Autodesk Inventor part; units mm, degrees
(part 2 of 2)
sketch "Block3" plane through (0, 0, 0) normal (0, 0, 1) x (1, 0, 0)
  spline S0 degree 3 poles (512.2411, -949.0199) (482.4419, -902.9014) (466.6908, -849.3536) (466.6908, -794.1657) (466.6908, -740.4054) (481.691, -688.0364) (510.0715, -642.7215) (519.4139, -627.8019) (514.8946, -608.1328) (499.9744, -598.7885) (485.0506, -589.4424) (465.3833, -593.9635) (456.0413, -608.886) (421.3023, -664.3538) (402.9407, -728.4231) (402.9407, -794.1657) (402.9407, -861.6551) (422.2206, -927.1657) (458.697, -983.6183) (464.796, -993.0562) (475.039, -998.198) (485.4977, -998.198) (491.424, -998.198) (497.42, -996.5464) (502.768, -993.091) (517.5543, -983.5387) (521.7951, -963.8054) (512.2411, -949.0199) knots 0 0 0 0 1 1 1 2 2 2 3 3 3 4 4 4 5 5 5 6 6 6 7 7 7 8 8 8 9 9 9 9
  line L0 (512.2411, -949.0199) -> (482.4419, -902.9014) construction
  line L1 (482.4419, -902.9014) -> (466.6908, -849.3536) construction
  line L2 (466.6908, -849.3536) -> (466.6908, -794.1657) construction
  line L3 (466.6908, -794.1657) -> (466.6908, -740.4054) construction
  line L4 (466.6908, -740.4054) -> (481.691, -688.0364) construction
  line L5 (481.691, -688.0364) -> (510.0715, -642.7215) construction
  line L6 (510.0715, -642.7215) -> (519.4139, -627.8019) construction
  line L7 (519.4139, -627.8019) -> (514.8946, -608.1328) construction
  line L8 (514.8946, -608.1328) -> (499.9744, -598.7885) construction
  line L9 (499.9744, -598.7885) -> (485.0506, -589.4424) construction
  line L10 (485.0506, -589.4424) -> (465.3833, -593.9635) construction
  line L11 (465.3833, -593.9635) -> (456.0413, -608.886) construction
  line L12 (456.0413, -608.886) -> (421.3023, -664.3538) construction
  line L13 (421.3023, -664.3538) -> (402.9407, -728.4231) construction
  line L14 (402.9407, -728.4231) -> (402.9407, -794.1657) construction
  line L15 (402.9407, -794.1657) -> (402.9407, -861.6551) construction
  line L16 (402.9407, -861.6551) -> (422.2206, -927.1657) construction
  line L17 (422.2206, -927.1657) -> (458.697, -983.6183) construction
  line L18 (458.697, -983.6183) -> (464.796, -993.0562) construction
  line L19 (464.796, -993.0562) -> (475.039, -998.198) construction
  line L20 (475.039, -998.198) -> (485.4977, -998.198) construction
  line L21 (485.4977, -998.198) -> (491.424, -998.198) construction
  line L22 (491.424, -998.198) -> (497.42, -996.5464) construction
  line L23 (497.42, -996.5464) -> (502.768, -993.091) construction
  line L24 (502.768, -993.091) -> (517.5543, -983.5387) construction
  line L25 (517.5543, -983.5387) -> (521.7951, -963.8054) construction
  line L26 (521.7951, -963.8054) -> (512.2411, -949.0199) construction
  spline S1 degree 3 poles (319.2882, -794.1657) (319.2882, -712.6801) (342.0267, -633.2978) (385.0462, -564.6002) (394.9736, -548.7483) (390.1703, -527.8498) (374.3166, -517.9219) (358.4587, -507.988) (337.5639, -512.8013) (327.6383, -528.651) (277.8625, -608.1368) (251.5537, -699.9486) (251.5537, -794.1657) (251.5537, -890.8995) (279.1817, -984.7874) (331.4532, -1065.6794) (337.9337, -1075.7068) (348.8188, -1081.1697) (359.9295, -1081.1697) (366.2274, -1081.1697) (372.5968, -1079.4151) (378.2798, -1075.7439) (393.9893, -1065.5921) (398.4951, -1044.6277) (388.3438, -1028.9177) (343.1674, -959.0039) (319.2882, -877.8281) (319.2882, -794.1657) knots 0 0 0 0 1 1 1 2 2 2 3 3 3 4 4 4 5 5 5 6 6 6 7 7 7 8 8 8 9 9 9 9
  line L27 (319.2882, -794.1657) -> (319.2882, -712.6801) construction
  line L28 (319.2882, -712.6801) -> (342.0267, -633.2978) construction
  line L29 (342.0267, -633.2978) -> (385.0462, -564.6002) construction
  line L30 (385.0462, -564.6002) -> (394.9736, -548.7483) construction
  line L31 (394.9736, -548.7483) -> (390.1703, -527.8498) construction
  line L32 (390.1703, -527.8498) -> (374.3166, -517.9219) construction
  line L33 (374.3166, -517.9219) -> (358.4587, -507.988) construction
  line L34 (358.4587, -507.988) -> (337.5639, -512.8013) construction
  line L35 (337.5639, -512.8013) -> (327.6383, -528.651) construction
  line L36 (327.6383, -528.651) -> (277.8625, -608.1368) construction
  line L37 (277.8625, -608.1368) -> (251.5537, -699.9486) construction
  line L38 (251.5537, -699.9486) -> (251.5537, -794.1657) construction
  line L39 (251.5537, -794.1657) -> (251.5537, -890.8995) construction
  line L40 (251.5537, -890.8995) -> (279.1817, -984.7874) construction
  line L41 (279.1817, -984.7874) -> (331.4532, -1065.6794) construction
  line L42 (331.4532, -1065.6794) -> (337.9337, -1075.7068) construction
  line L43 (337.9337, -1075.7068) -> (348.8188, -1081.1697) construction
  line L44 (348.8188, -1081.1697) -> (359.9295, -1081.1697) construction
  line L45 (359.9295, -1081.1697) -> (366.2274, -1081.1697) construction
  line L46 (366.2274, -1081.1697) -> (372.5968, -1079.4151) construction
  line L47 (372.5968, -1079.4151) -> (378.2798, -1075.7439) construction
  line L48 (378.2798, -1075.7439) -> (393.9893, -1065.5921) construction
  line L49 (393.9893, -1065.5921) -> (398.4951, -1044.6277) construction
  line L50 (398.4951, -1044.6277) -> (388.3438, -1028.9177) construction
  line L51 (388.3438, -1028.9177) -> (343.1674, -959.0039) construction
  line L52 (343.1674, -959.0039) -> (319.2882, -877.8281) construction
  line L53 (319.2882, -877.8281) -> (319.2882, -794.1657) construction
  spline S2 degree 3 poles (1624.0756, -517.9219) (1608.2155, -527.8479) (1603.4145, -548.7464) (1613.3442, -564.6002) (1656.3632, -633.3018) (1679.1022, -712.6859) (1679.1022, -794.1657) (1679.1022, -877.824) (1655.2189, -958.9999) (1610.0371, -1028.9177) (1599.889, -1044.6277) (1604.3952, -1065.5921) (1620.1065, -1075.7439) (1625.7877, -1079.4168) (1632.1535, -1081.1697) (1638.4568, -1081.1697) (1649.5617, -1081.1697) (1660.4485, -1075.7068) (1666.9313, -1065.6794) (1719.2028, -984.7839) (1746.8372, -890.896) (1746.8372, -794.1657) (1746.8372, -699.9567) (1720.5256, -608.1423) (1670.7521, -528.651) (1660.8224, -512.799) (1639.9199, -507.9958) (1624.0756, -517.9219) knots 0 0 0 0 1 1 1 2 2 2 3 3 3 4 4 4 5 5 5 6 6 6 7 7 7 8 8 8 9 9 9 9
  line L54 (1624.0756, -517.9219) -> (1608.2155, -527.8479) construction
  line L55 (1608.2155, -527.8479) -> (1603.4145, -548.7464) construction
  line L56 (1603.4145, -548.7464) -> (1613.3442, -564.6002) construction
  line L57 (1613.3442, -564.6002) -> (1656.3632, -633.3018) construction
  line L58 (1656.3632, -633.3018) -> (1679.1022, -712.6859) construction
  line L59 (1679.1022, -712.6859) -> (1679.1022, -794.1657) construction
  line L60 (1679.1022, -794.1657) -> (1679.1022, -877.824) construction
  line L61 (1679.1022, -877.824) -> (1655.2189, -958.9999) construction
  line L62 (1655.2189, -958.9999) -> (1610.0371, -1028.9177) construction
  line L63 (1610.0371, -1028.9177) -> (1599.889, -1044.6277) construction
  line L64 (1599.889, -1044.6277) -> (1604.3952, -1065.5921) construction
  line L65 (1604.3952, -1065.5921) -> (1620.1065, -1075.7439) construction
  line L66 (1620.1065, -1075.7439) -> (1625.7877, -1079.4168) construction
  line L67 (1625.7877, -1079.4168) -> (1632.1535, -1081.1697) construction
  line L68 (1632.1535, -1081.1697) -> (1638.4568, -1081.1697) construction
  line L69 (1638.4568, -1081.1697) -> (1649.5617, -1081.1697) construction
  line L70 (1649.5617, -1081.1697) -> (1660.4485, -1075.7068) construction
  line L71 (1660.4485, -1075.7068) -> (1666.9313, -1065.6794) construction
  line L72 (1666.9313, -1065.6794) -> (1719.2028, -984.7839) construction
  line L73 (1719.2028, -984.7839) -> (1746.8372, -890.896) construction
  line L74 (1746.8372, -890.896) -> (1746.8372, -794.1657) construction
  line L75 (1746.8372, -794.1657) -> (1746.8372, -699.9567) construction
  line L76 (1746.8372, -699.9567) -> (1720.5256, -608.1423) construction
  line L77 (1720.5256, -608.1423) -> (1670.7521, -528.651) construction
  line L78 (1670.7521, -528.651) -> (1660.8224, -512.799) construction
  line L79 (1660.8224, -512.799) -> (1639.9199, -507.9958) construction
  line L80 (1639.9199, -507.9958) -> (1624.0756, -517.9219) construction
  spline S3 degree 3 poles (1498.4042, -598.7908) (1483.4859, -608.1345) (1478.972, -627.8037) (1488.3109, -642.7238) (1516.6917, -688.0323) (1531.6955, -740.3996) (1531.6955, -794.1657) (1531.6955, -849.3514) (1515.9444, -902.8996) (1486.1474, -949.0213) (1476.5912, -963.8077) (1480.832, -983.5387) (1495.6255, -993.0932) (1500.9718, -996.5482) (1506.9641, -998.198) (1512.8862, -998.198) (1523.3454, -998.198) (1533.5939, -993.0539) (1539.6952, -983.6165) (1576.1617, -927.1639) (1595.4456, -861.6511) (1595.4456, -794.1657) (1595.4456, -728.4176) (1577.0799, -664.3461) (1542.3409, -608.8837) (1532.9948, -593.9635) (1513.3221, -589.4407) (1498.4042, -598.7908) knots 0 0 0 0 1 1 1 2 2 2 3 3 3 4 4 4 5 5 5 6 6 6 7 7 7 8 8 8 9 9 9 9
  line L81 (1498.4042, -598.7908) -> (1483.4859, -608.1345) construction
  line L82 (1483.4859, -608.1345) -> (1478.972, -627.8037) construction
  line L83 (1478.972, -627.8037) -> (1488.3109, -642.7238) construction
  line L84 (1488.3109, -642.7238) -> (1516.6917, -688.0323) construction
  line L85 (1516.6917, -688.0323) -> (1531.6955, -740.3996) construction
  line L86 (1531.6955, -740.3996) -> (1531.6955, -794.1657) construction
  line L87 (1531.6955, -794.1657) -> (1531.6955, -849.3514) construction
  line L88 (1531.6955, -849.3514) -> (1515.9444, -902.8996) construction
  line L89 (1515.9444, -902.8996) -> (1486.1474, -949.0213) construction
  line L90 (1486.1474, -949.0213) -> (1476.5912, -963.8077) construction
  line L91 (1476.5912, -963.8077) -> (1480.832, -983.5387) construction
  line L92 (1480.832, -983.5387) -> (1495.6255, -993.0932) construction
  line L93 (1495.6255, -993.0932) -> (1500.9718, -996.5482) construction
  line L94 (1500.9718, -996.5482) -> (1506.9641, -998.198) construction
  line L95 (1506.9641, -998.198) -> (1512.8862, -998.198) construction
  line L96 (1512.8862, -998.198) -> (1523.3454, -998.198) construction
  line L97 (1523.3454, -998.198) -> (1533.5939, -993.0539) construction
  line L98 (1533.5939, -993.0539) -> (1539.6952, -983.6165) construction
  line L99 (1539.6952, -983.6165) -> (1576.1617, -927.1639) construction
  line L100 (1576.1617, -927.1639) -> (1595.4456, -861.6511) construction
  line L101 (1595.4456, -861.6511) -> (1595.4456, -794.1657) construction
  line L102 (1595.4456, -794.1657) -> (1595.4456, -728.4176) construction
  line L103 (1595.4456, -728.4176) -> (1577.0799, -664.3461) construction
  line L104 (1577.0799, -664.3461) -> (1542.3409, -608.8837) construction
  line L105 (1542.3409, -608.8837) -> (1532.9948, -593.9635) construction
  line L106 (1532.9948, -593.9635) -> (1513.3221, -589.4407) construction
  line L107 (1513.3221, -589.4407) -> (1498.4042, -598.7908) construction
  point P0 (932.5278, -1154.2968)
sketch "Block4" plane through (0, 0, 0) normal (0, 0, 1) x (1, 0, 0)
  line L0 (-5.463, -3.5621) -> (5.8608, -3.5621)
  line L1 (5.8608, -3.5621) -> (5.8608, -2.6376)
  line L2 (5.8608, -2.6376) -> (4.5507, -1.3269) construction
  line L3 (4.5507, -1.3269) -> (4.5507, 1.5979)
  line L4 (4.5507, 1.5979) -> (1.1958, 5.8325) construction
  line L5 (1.1958, 5.8325) -> (0.2099, 6.8188) construction
  line L6 (0.2099, 6.8188) -> (-0.7872, 5.822) construction
  line L7 (-0.7872, 5.822) -> (-4.1524, 1.5979) construction
  line L8 (-4.1524, 1.5979) -> (-4.1524, -1.3271)
  line L9 (-4.1524, -1.3271) -> (-5.463, -2.6376) construction
  line L10 (-5.463, -2.6376) -> (-5.463, -3.5621)
  line L11 (2.0223, -4.3362) -> (0.2001, -5.717) construction
  line L12 (0.2001, -5.717) -> (-1.6247, -4.3362) construction
  arc A0 (5.8608, -2.6376) -> (4.5507, -1.3269) centre (4.5502, -2.6376) ccw
  arc A1 (-4.1524, -1.3271) -> (-5.463, -2.6376) centre (-4.1526, -2.6376) ccw
  arc A2 (-1.6247, -4.3362) -> (2.0223, -4.3362) centre (0.1988, -3.8225) ccw
  arc A3 (1.1958, 5.8325) -> (-0.7872, 5.822) centre (0.2043, 5.8273) ccw
  arc A4 (-0.7872, 5.822) -> (-4.1524, 1.5979) centre (0.1814, 1.5979) ccw
  arc A5 (4.5507, 1.5979) -> (1.1958, 5.8325) centre (0.2008, 1.5979) ccw
  spline S0 degree 3 poles (-9.91, 1.6654) (-9.91, 2.8877) (-9.5689, 4.0784) (-8.9236, 5.1089) (-8.7747, 5.3466) (-8.8468, 5.6601) (-9.0846, 5.809) (-9.3224, 5.958) (-9.6359, 5.8858) (-9.7848, 5.6481) (-10.5314, 4.4558) (-10.926, 3.0786) (-10.926, 1.6654) (-10.926, 0.2144) (-10.5116, -1.194) (-9.7275, -2.4073) (-9.6303, -2.5577) (-9.467, -2.6397) (-9.3004, -2.6397) (-9.2059, -2.6397) (-9.1104, -2.6134) (-9.0251, -2.5583) (-8.7895, -2.406) (-8.7219, -2.0916) (-8.8742, -1.8559) (-9.5518, -0.8072) (-9.91, 0.4104) (-9.91, 1.6654) knots 0 0 0 0 1 1 1 2 2 2 3 3 3 4 4 4 5 5 5 6 6 6 7 7 7 8 8 8 9 9 9 9
  line L13 (-9.91, 1.6654) -> (-9.91, 2.8877) construction
  line L14 (-9.91, 2.8877) -> (-9.5689, 4.0784) construction
  line L15 (-9.5689, 4.0784) -> (-8.9236, 5.1089) construction
  line L16 (-8.9236, 5.1089) -> (-8.7747, 5.3466) construction
  line L17 (-8.7747, 5.3466) -> (-8.8468, 5.6601) construction
  line L18 (-8.8468, 5.6601) -> (-9.0846, 5.809) construction
  line L19 (-9.0846, 5.809) -> (-9.3224, 5.958) construction
  line L20 (-9.3224, 5.958) -> (-9.6359, 5.8858) construction
  line L21 (-9.6359, 5.8858) -> (-9.7848, 5.6481) construction
  line L22 (-9.7848, 5.6481) -> (-10.5314, 4.4558) construction
  line L23 (-10.5314, 4.4558) -> (-10.926, 3.0786) construction
  line L24 (-10.926, 3.0786) -> (-10.926, 1.6654) construction
  line L25 (-10.926, 1.6654) -> (-10.926, 0.2144) construction
  line L26 (-10.926, 0.2144) -> (-10.5116, -1.194) construction
  line L27 (-10.5116, -1.194) -> (-9.7275, -2.4073) construction
  line L28 (-9.7275, -2.4073) -> (-9.6303, -2.5577) construction
  line L29 (-9.6303, -2.5577) -> (-9.467, -2.6397) construction
  line L30 (-9.467, -2.6397) -> (-9.3004, -2.6397) construction
  line L31 (-9.3004, -2.6397) -> (-9.2059, -2.6397) construction
  line L32 (-9.2059, -2.6397) -> (-9.1104, -2.6134) construction
  line L33 (-9.1104, -2.6134) -> (-9.0251, -2.5583) construction
  line L34 (-9.0251, -2.5583) -> (-8.7895, -2.406) construction
  line L35 (-8.7895, -2.406) -> (-8.7219, -2.0916) construction
  line L36 (-8.7219, -2.0916) -> (-8.8742, -1.8559) construction
  line L37 (-8.8742, -1.8559) -> (-9.5518, -0.8072) construction
  line L38 (-9.5518, -0.8072) -> (-9.91, 0.4104) construction
  line L39 (-9.91, 0.4104) -> (-9.91, 1.6654) construction
  spline S1 degree 3 poles (9.6618, 5.809) (9.4239, 5.6601) (9.3519, 5.3467) (9.5008, 5.1089) (10.1461, 4.0783) (10.4872, 2.8876) (10.4872, 1.6654) (10.4872, 0.4105) (10.129, -0.8071) (9.4512, -1.8559) (9.299, -2.0916) (9.3666, -2.406) (9.6023, -2.5583) (9.6875, -2.6134) (9.783, -2.6397) (9.8775, -2.6397) (10.0441, -2.6397) (10.2074, -2.5577) (10.3046, -2.4073) (11.0887, -1.1939) (11.5032, 0.2144) (11.5032, 1.6654) (11.5032, 3.0785) (11.1086, 4.4557) (10.362, 5.6481) (10.213, 5.8859) (9.8995, 5.9579) (9.6618, 5.809) knots 0 0 0 0 1 1 1 2 2 2 3 3 3 4 4 4 5 5 5 6 6 6 7 7 7 8 8 8 9 9 9 9
  line L40 (9.6618, 5.809) -> (9.4239, 5.6601) construction
  line L41 (9.4239, 5.6601) -> (9.3519, 5.3467) construction
  line L42 (9.3519, 5.3467) -> (9.5008, 5.1089) construction
  line L43 (9.5008, 5.1089) -> (10.1461, 4.0783) construction
  line L44 (10.1461, 4.0783) -> (10.4872, 2.8876) construction
  line L45 (10.4872, 2.8876) -> (10.4872, 1.6654) construction
  line L46 (10.4872, 1.6654) -> (10.4872, 0.4105) construction
  line L47 (10.4872, 0.4105) -> (10.129, -0.8071) construction
  line L48 (10.129, -0.8071) -> (9.4512, -1.8559) construction
  line L49 (9.4512, -1.8559) -> (9.299, -2.0916) construction
  line L50 (9.299, -2.0916) -> (9.3666, -2.406) construction
  line L51 (9.3666, -2.406) -> (9.6023, -2.5583) construction
  line L52 (9.6023, -2.5583) -> (9.6875, -2.6134) construction
  line L53 (9.6875, -2.6134) -> (9.783, -2.6397) construction
  line L54 (9.783, -2.6397) -> (9.8775, -2.6397) construction
  line L55 (9.8775, -2.6397) -> (10.0441, -2.6397) construction
  line L56 (10.0441, -2.6397) -> (10.2074, -2.5577) construction
  line L57 (10.2074, -2.5577) -> (10.3046, -2.4073) construction
  line L58 (10.3046, -2.4073) -> (11.0887, -1.1939) construction
  line L59 (11.0887, -1.1939) -> (11.5032, 0.2144) construction
  line L60 (11.5032, 0.2144) -> (11.5032, 1.6654) construction
  line L61 (11.5032, 1.6654) -> (11.5032, 3.0785) construction
  line L62 (11.5032, 3.0785) -> (11.1086, 4.4557) construction
  line L63 (11.1086, 4.4557) -> (10.362, 5.6481) construction
  line L64 (10.362, 5.6481) -> (10.213, 5.8859) construction
  line L65 (10.213, 5.8859) -> (9.8995, 5.9579) construction
  line L66 (9.8995, 5.9579) -> (9.6618, 5.809) construction
  spline S2 degree 3 poles (7.7767, 4.596) (7.553, 4.4558) (7.4852, 4.1608) (7.6253, 3.937) (8.051, 3.2574) (8.2761, 2.4719) (8.2761, 1.6654) (8.2761, 0.8376) (8.0398, 0.0344) (7.5929, -0.6575) (7.4495, -0.8793) (7.5131, -1.1752) (7.7351, -1.3185) (7.8152, -1.3704) (7.9051, -1.3951) (7.994, -1.3951) (8.1509, -1.3951) (8.3046, -1.318) (8.3961, -1.1764) (8.9431, -0.3296) (9.2324, 0.6531) (9.2324, 1.6654) (9.2324, 2.6516) (8.9569, 3.6127) (8.4358, 4.4446) (8.2956, 4.6684) (8.0005, 4.7362) (7.7767, 4.596) knots 0 0 0 0 1 1 1 2 2 2 3 3 3 4 4 4 5 5 5 6 6 6 7 7 7 8 8 8 9 9 9 9
  line L67 (7.7767, 4.596) -> (7.553, 4.4558) construction
  line L68 (7.553, 4.4558) -> (7.4852, 4.1608) construction
  line L69 (7.4852, 4.1608) -> (7.6253, 3.937) construction
  line L70 (7.6253, 3.937) -> (8.051, 3.2574) construction
  line L71 (8.051, 3.2574) -> (8.2761, 2.4719) construction
  line L72 (8.2761, 2.4719) -> (8.2761, 1.6654) construction
  line L73 (8.2761, 1.6654) -> (8.2761, 0.8376) construction
  line L74 (8.2761, 0.8376) -> (8.0398, 0.0344) construction
  line L75 (8.0398, 0.0344) -> (7.5929, -0.6575) construction
  line L76 (7.5929, -0.6575) -> (7.4495, -0.8793) construction
  line L77 (7.4495, -0.8793) -> (7.5131, -1.1752) construction
  line L78 (7.5131, -1.1752) -> (7.7351, -1.3185) construction
  line L79 (7.7351, -1.3185) -> (7.8152, -1.3704) construction
  line L80 (7.8152, -1.3704) -> (7.9051, -1.3951) construction
  line L81 (7.9051, -1.3951) -> (7.994, -1.3951) construction
  line L82 (7.994, -1.3951) -> (8.1509, -1.3951) construction
  line L83 (8.1509, -1.3951) -> (8.3046, -1.318) construction
  line L84 (8.3046, -1.318) -> (8.3961, -1.1764) construction
  line L85 (8.3961, -1.1764) -> (8.9431, -0.3296) construction
  line L86 (8.9431, -0.3296) -> (9.2324, 0.6531) construction
  line L87 (9.2324, 0.6531) -> (9.2324, 1.6654) construction
  line L88 (9.2324, 1.6654) -> (9.2324, 2.6516) construction
  line L89 (9.2324, 2.6516) -> (8.9569, 3.6127) construction
  line L90 (8.9569, 3.6127) -> (8.4358, 4.4446) construction
  line L91 (8.4358, 4.4446) -> (8.2956, 4.6684) construction
  line L92 (8.2956, 4.6684) -> (8.0005, 4.7362) construction
  line L93 (8.0005, 4.7362) -> (7.7767, 4.596) construction
  spline S3 degree 3 poles (-7.0157, -0.6574) (-7.4627, 0.0343) (-7.699, 0.8376) (-7.699, 1.6654) (-7.699, 2.4718) (-7.474, 3.2573) (-7.0483, 3.937) (-6.9081, 4.1608) (-6.9759, 4.4559) (-7.1997, 4.596) (-7.4236, 4.7362) (-7.7186, 4.6684) (-7.8587, 4.4446) (-8.3798, 3.6125) (-8.6552, 2.6515) (-8.6552, 1.6654) (-8.6552, 0.653) (-8.366, -0.3296) (-7.8189, -1.1764) (-7.7274, -1.318) (-7.5737, -1.3951) (-7.4169, -1.3951) (-7.328, -1.3951) (-7.238, -1.3703) (-7.1578, -1.3185) (-6.936, -1.1752) (-6.8724, -0.8792) (-7.0157, -0.6574) knots 0 0 0 0 1 1 1 2 2 2 3 3 3 4 4 4 5 5 5 6 6 6 7 7 7 8 8 8 9 9 9 9
  line L94 (-7.0157, -0.6574) -> (-7.4627, 0.0343) construction
  line L95 (-7.4627, 0.0343) -> (-7.699, 0.8376) construction
  line L96 (-7.699, 0.8376) -> (-7.699, 1.6654) construction
  line L97 (-7.699, 1.6654) -> (-7.699, 2.4718) construction
  line L98 (-7.699, 2.4718) -> (-7.474, 3.2573) construction
  line L99 (-7.474, 3.2573) -> (-7.0483, 3.937) construction
  line L100 (-7.0483, 3.937) -> (-6.9081, 4.1608) construction
  line L101 (-6.9081, 4.1608) -> (-6.9759, 4.4559) construction
  line L102 (-6.9759, 4.4559) -> (-7.1997, 4.596) construction
  line L103 (-7.1997, 4.596) -> (-7.4236, 4.7362) construction
  line L104 (-7.4236, 4.7362) -> (-7.7186, 4.6684) construction
  line L105 (-7.7186, 4.6684) -> (-7.8587, 4.4446) construction
  line L106 (-7.8587, 4.4446) -> (-8.3798, 3.6125) construction
  line L107 (-8.3798, 3.6125) -> (-8.6552, 2.6515) construction
  line L108 (-8.6552, 2.6515) -> (-8.6552, 1.6654) construction
  line L109 (-8.6552, 1.6654) -> (-8.6552, 0.653) construction
  line L110 (-8.6552, 0.653) -> (-8.366, -0.3296) construction
  line L111 (-8.366, -0.3296) -> (-7.8189, -1.1764) construction
  line L112 (-7.8189, -1.1764) -> (-7.7274, -1.318) construction
  line L113 (-7.7274, -1.318) -> (-7.5737, -1.3951) construction
  line L114 (-7.5737, -1.3951) -> (-7.4169, -1.3951) construction
  line L115 (-7.4169, -1.3951) -> (-7.328, -1.3951) construction
  line L116 (-7.328, -1.3951) -> (-7.238, -1.3703) construction
  line L117 (-7.238, -1.3703) -> (-7.1578, -1.3185) construction
  line L118 (-7.1578, -1.3185) -> (-6.936, -1.1752) construction
  line L119 (-6.936, -1.1752) -> (-6.8724, -0.8792) construction
  line L120 (-6.8724, -0.8792) -> (-7.0157, -0.6574) construction
  line L121 (-1.6247, -4.3362) -> (2.0223, -4.3362)
  point P0 (0.2378, 1.0132)
sketch "Sketch1" plane through (0, 0, 0) normal (0, 0, 1) x (1, 0, 0)
  line L0 (-45.15, -44.25) -> (45.15, -44.25)
  line L1 (45.15, -44.25) -> (45.15, 44.25)
  line L2 (45.15, 44.25) -> (-45.15, 44.25)
  line L3 (-45.15, 44.25) -> (-45.15, -44.25)
  line L4 (-45.15, -44.25) -> (45.15, 44.25) construction
  line L5 (45.15, -44.25) -> (-45.15, 44.25) construction
  point P0 (0, 0)
  dimension "d0" = 90.3
  dimension "d1" = 88.5
  constraints: 12 end point, 2 midpoint, 2 parallel, 1 horizontal, 1 perpendicular
  measures "d0" distance of L2.end L1.end
  measures "d1" distance of L1.end L0.end
extrude "Extrusion1" add sketch "Sketch1" along normal blind 3
sketch "Sketch2" plane through (0, 0, 3) normal (0, 0, 1) x (1, 0, 0)
  line L0 (0, 0) -> (4.3515, 0) construction
  line L1 (0, 0) -> (-4.3515, 0) construction
  line L2 (-5.6622, -4.2334) -> (5.6617, -4.2334)
  line L3 (5.6617, -4.2334) -> (5.6617, -3.3088)
  line L4 (5.6617, -3.3088) -> (4.3515, -1.9981) construction
  line L5 (4.3515, -1.9981) -> (4.3515, 0.9267)
  line L6 (4.3515, 0.9267) -> (0.9967, 5.1613) construction
  line L7 (0.9967, 5.1613) -> (0.0108, 6.1476) construction
  line L8 (0.0108, 6.1476) -> (-0.9864, 5.1508) construction
  line L9 (-0.9864, 5.1508) -> (-4.3515, 0.9267) construction
  line L10 (-4.3515, 0.9267) -> (-4.3515, -1.9984)
  line L11 (-4.3515, -1.9984) -> (-5.6622, -3.3088) construction
  line L12 (-5.6622, -3.3088) -> (-5.6622, -4.2334)
  line L13 (1.8231, -5.0075) -> (0.001, -6.3882) construction
  line L14 (0.001, -6.3882) -> (-1.8239, -5.0075) construction
  arc A0 (5.6617, -3.3088) -> (4.3515, -1.9981) centre (4.351, -3.3088) ccw
  arc A1 (-4.3515, -1.9984) -> (-5.6622, -3.3088) centre (-4.3518, -3.3088) ccw
  arc A2 (-1.8239, -5.0075) -> (1.8231, -5.0075) centre (-0.0004, -4.4937) ccw
  arc A3 (0.9967, 5.1613) -> (-0.9864, 5.1508) centre (0.0051, 5.156) ccw
  arc A4 (-0.9864, 5.1508) -> (-4.3515, 0.9267) centre (-0.0178, 0.9267) ccw
  arc A5 (4.3515, 0.9267) -> (0.9967, 5.1613) centre (0.0016, 0.9267) ccw
  spline S0 degree 3 poles (-10.1092, 0.9941) (-10.1092, 2.2164) (-9.7681, 3.4072) (-9.1228, 4.4376) (-8.9739, 4.6754) (-9.0459, 4.9889) (-9.2837, 5.1378) (-9.5216, 5.2868) (-9.835, 5.2146) (-9.9839, 4.9769) (-10.7306, 3.7846) (-11.1252, 2.4074) (-11.1252, 0.9941) (-11.1252, -0.4569) (-10.7108, -1.8652) (-9.9267, -3.0786) (-9.8295, -3.229) (-9.6662, -3.3109) (-9.4996, -3.3109) (-9.4051, -3.3109) (-9.3095, -3.2846) (-9.2243, -3.2295) (-8.9887, -3.0773) (-8.9211, -2.7628) (-9.0733, -2.5271) (-9.751, -1.4784) (-10.1092, -0.2608) (-10.1092, 0.9941) knots 0 0 0 0 1 1 1 2 2 2 3 3 3 4 4 4 5 5 5 6 6 6 7 7 7 8 8 8 9 9 9 9
  line L15 (-10.1092, 0.9941) -> (-10.1092, 2.2164) construction
  line L16 (-10.1092, 2.2164) -> (-9.7681, 3.4072) construction
  line L17 (-9.7681, 3.4072) -> (-9.1228, 4.4376) construction
  line L18 (-9.1228, 4.4376) -> (-8.9739, 4.6754) construction
  line L19 (-8.9739, 4.6754) -> (-9.0459, 4.9889) construction
  line L20 (-9.0459, 4.9889) -> (-9.2837, 5.1378) construction
  line L21 (-9.2837, 5.1378) -> (-9.5216, 5.2868) construction
  line L22 (-9.5216, 5.2868) -> (-9.835, 5.2146) construction
  line L23 (-9.835, 5.2146) -> (-9.9839, 4.9769) construction
  line L24 (-9.9839, 4.9769) -> (-10.7306, 3.7846) construction
  line L25 (-10.7306, 3.7846) -> (-11.1252, 2.4074) construction
  line L26 (-11.1252, 2.4074) -> (-11.1252, 0.9941) construction
  line L27 (-11.1252, 0.9941) -> (-11.1252, -0.4569) construction
  line L28 (-11.1252, -0.4569) -> (-10.7108, -1.8652) construction
  line L29 (-10.7108, -1.8652) -> (-9.9267, -3.0786) construction
  line L30 (-9.9267, -3.0786) -> (-9.8295, -3.229) construction
  line L31 (-9.8295, -3.229) -> (-9.6662, -3.3109) construction
  line L32 (-9.6662, -3.3109) -> (-9.4996, -3.3109) construction
  line L33 (-9.4996, -3.3109) -> (-9.4051, -3.3109) construction
  line L34 (-9.4051, -3.3109) -> (-9.3095, -3.2846) construction
  line L35 (-9.3095, -3.2846) -> (-9.2243, -3.2295) construction
  line L36 (-9.2243, -3.2295) -> (-8.9887, -3.0773) construction
  line L37 (-8.9887, -3.0773) -> (-8.9211, -2.7628) construction
  line L38 (-8.9211, -2.7628) -> (-9.0733, -2.5271) construction
  line L39 (-9.0733, -2.5271) -> (-9.751, -1.4784) construction
  line L40 (-9.751, -1.4784) -> (-10.1092, -0.2608) construction
  line L41 (-10.1092, -0.2608) -> (-10.1092, 0.9941) construction
  spline S1 degree 3 poles (9.4626, 5.1378) (9.2247, 4.9889) (9.1527, 4.6754) (9.3017, 4.4376) (9.947, 3.4071) (10.288, 2.2163) (10.288, 0.9941) (10.288, -0.2607) (9.9298, -1.4784) (9.2521, -2.5271) (9.0998, -2.7628) (9.1674, -3.0773) (9.4031, -3.2295) (9.4883, -3.2846) (9.5838, -3.3109) (9.6784, -3.3109) (9.8449, -3.3109) (10.0082, -3.229) (10.1055, -3.0786) (10.8895, -1.8651) (11.3041, -0.4568) (11.3041, 0.9941) (11.3041, 2.4073) (10.9094, 3.7845) (10.1628, 4.9769) (10.0138, 5.2146) (9.7003, 5.2867) (9.4626, 5.1378) knots 0 0 0 0 1 1 1 2 2 2 3 3 3 4 4 4 5 5 5 6 6 6 7 7 7 8 8 8 9 9 9 9
  line L42 (9.4626, 5.1378) -> (9.2247, 4.9889) construction
  line L43 (9.2247, 4.9889) -> (9.1527, 4.6754) construction
  line L44 (9.1527, 4.6754) -> (9.3017, 4.4376) construction
  line L45 (9.3017, 4.4376) -> (9.947, 3.4071) construction
  line L46 (9.947, 3.4071) -> (10.288, 2.2163) construction
  line L47 (10.288, 2.2163) -> (10.288, 0.9941) construction
  line L48 (10.288, 0.9941) -> (10.288, -0.2607) construction
  line L49 (10.288, -0.2607) -> (9.9298, -1.4784) construction
  line L50 (9.9298, -1.4784) -> (9.2521, -2.5271) construction
  line L51 (9.2521, -2.5271) -> (9.0998, -2.7628) construction
  line L52 (9.0998, -2.7628) -> (9.1674, -3.0773) construction
  line L53 (9.1674, -3.0773) -> (9.4031, -3.2295) construction
  line L54 (9.4031, -3.2295) -> (9.4883, -3.2846) construction
  line L55 (9.4883, -3.2846) -> (9.5838, -3.3109) construction
  line L56 (9.5838, -3.3109) -> (9.6784, -3.3109) construction
  line L57 (9.6784, -3.3109) -> (9.8449, -3.3109) construction
  line L58 (9.8449, -3.3109) -> (10.0082, -3.229) construction
  line L59 (10.0082, -3.229) -> (10.1055, -3.0786) construction
  line L60 (10.1055, -3.0786) -> (10.8895, -1.8651) construction
  line L61 (10.8895, -1.8651) -> (11.3041, -0.4568) construction
  line L62 (11.3041, -0.4568) -> (11.3041, 0.9941) construction
  line L63 (11.3041, 0.9941) -> (11.3041, 2.4073) construction
  line L64 (11.3041, 2.4073) -> (10.9094, 3.7845) construction
  line L65 (10.9094, 3.7845) -> (10.1628, 4.9769) construction
  line L66 (10.1628, 4.9769) -> (10.0138, 5.2146) construction
  line L67 (10.0138, 5.2146) -> (9.7003, 5.2867) construction
  line L68 (9.7003, 5.2867) -> (9.4626, 5.1378) construction
  spline S2 degree 3 poles (7.5776, 3.9248) (7.3538, 3.7846) (7.2861, 3.4896) (7.4262, 3.2658) (7.8519, 2.5861) (8.0769, 1.8006) (8.0769, 0.9941) (8.0769, 0.1663) (7.8407, -0.6369) (7.3937, -1.3287) (7.2504, -1.5505) (7.314, -1.8465) (7.5359, -1.9898) (7.6161, -2.0416) (7.706, -2.0664) (7.7948, -2.0664) (7.9517, -2.0664) (8.1054, -1.9892) (8.1969, -1.8476) (8.7439, -1.0008) (9.0332, -0.0181) (9.0332, 0.9941) (9.0332, 1.9804) (8.7577, 2.9414) (8.2366, 3.7734) (8.0964, 3.9972) (7.8013, 4.065) (7.5776, 3.9248) knots 0 0 0 0 1 1 1 2 2 2 3 3 3 4 4 4 5 5 5 6 6 6 7 7 7 8 8 8 9 9 9 9
  line L69 (7.5776, 3.9248) -> (7.3538, 3.7846) construction
  line L70 (7.3538, 3.7846) -> (7.2861, 3.4896) construction
  line L71 (7.2861, 3.4896) -> (7.4262, 3.2658) construction
  line L72 (7.4262, 3.2658) -> (7.8519, 2.5861) construction
  line L73 (7.8519, 2.5861) -> (8.0769, 1.8006) construction
  line L74 (8.0769, 1.8006) -> (8.0769, 0.9941) construction
  line L75 (8.0769, 0.9941) -> (8.0769, 0.1663) construction
  line L76 (8.0769, 0.1663) -> (7.8407, -0.6369) construction
  line L77 (7.8407, -0.6369) -> (7.3937, -1.3287) construction
  line L78 (7.3937, -1.3287) -> (7.2504, -1.5505) construction
  line L79 (7.2504, -1.5505) -> (7.314, -1.8465) construction
  line L80 (7.314, -1.8465) -> (7.5359, -1.9898) construction
  line L81 (7.5359, -1.9898) -> (7.6161, -2.0416) construction
  line L82 (7.6161, -2.0416) -> (7.706, -2.0664) construction
  line L83 (7.706, -2.0664) -> (7.7948, -2.0664) construction
  line L84 (7.7948, -2.0664) -> (7.9517, -2.0664) construction
  line L85 (7.9517, -2.0664) -> (8.1054, -1.9892) construction
  line L86 (8.1054, -1.9892) -> (8.1969, -1.8476) construction
  line L87 (8.1969, -1.8476) -> (8.7439, -1.0008) construction
  line L88 (8.7439, -1.0008) -> (9.0332, -0.0181) construction
  line L89 (9.0332, -0.0181) -> (9.0332, 0.9941) construction
  line L90 (9.0332, 0.9941) -> (9.0332, 1.9804) construction
  line L91 (9.0332, 1.9804) -> (8.7577, 2.9414) construction
  line L92 (8.7577, 2.9414) -> (8.2366, 3.7734) construction
  line L93 (8.2366, 3.7734) -> (8.0964, 3.9972) construction
  line L94 (8.0964, 3.9972) -> (7.8013, 4.065) construction
  line L95 (7.8013, 4.065) -> (7.5776, 3.9248) construction
  spline S3 degree 3 poles (-7.2149, -1.3287) (-7.6619, -0.6369) (-7.8981, 0.1663) (-7.8981, 0.9941) (-7.8981, 1.8005) (-7.6731, 2.5861) (-7.2474, 3.2658) (-7.1073, 3.4896) (-7.1751, 3.7846) (-7.3989, 3.9248) (-7.6227, 4.065) (-7.9177, 3.9972) (-8.0579, 3.7733) (-8.579, 2.9413) (-8.8544, 1.9803) (-8.8544, 0.9941) (-8.8544, -0.0182) (-8.5652, -1.0009) (-8.018, -1.8477) (-7.9266, -1.9892) (-7.7729, -2.0664) (-7.616, -2.0664) (-7.5271, -2.0664) (-7.4372, -2.0416) (-7.357, -1.9897) (-7.1352, -1.8465) (-7.0716, -1.5505) (-7.2149, -1.3287) knots 0 0 0 0 1 1 1 2 2 2 3 3 3 4 4 4 5 5 5 6 6 6 7 7 7 8 8 8 9 9 9 9
  line L96 (-7.2149, -1.3287) -> (-7.6619, -0.6369) construction
  line L97 (-7.6619, -0.6369) -> (-7.8981, 0.1663) construction
  line L98 (-7.8981, 0.1663) -> (-7.8981, 0.9941) construction
  line L99 (-7.8981, 0.9941) -> (-7.8981, 1.8005) construction
  line L100 (-7.8981, 1.8005) -> (-7.6731, 2.5861) construction
  line L101 (-7.6731, 2.5861) -> (-7.2474, 3.2658) construction
  line L102 (-7.2474, 3.2658) -> (-7.1073, 3.4896) construction
  line L103 (-7.1073, 3.4896) -> (-7.1751, 3.7846) construction
  line L104 (-7.1751, 3.7846) -> (-7.3989, 3.9248) construction
  line L105 (-7.3989, 3.9248) -> (-7.6227, 4.065) construction
  line L106 (-7.6227, 4.065) -> (-7.9177, 3.9972) construction
  line L107 (-7.9177, 3.9972) -> (-8.0579, 3.7733) construction
  line L108 (-8.0579, 3.7733) -> (-8.579, 2.9413) construction
  line L109 (-8.579, 2.9413) -> (-8.8544, 1.9803) construction
  line L110 (-8.8544, 1.9803) -> (-8.8544, 0.9941) construction
  line L111 (-8.8544, 0.9941) -> (-8.8544, -0.0182) construction
  line L112 (-8.8544, -0.0182) -> (-8.5652, -1.0009) construction
  line L113 (-8.5652, -1.0009) -> (-8.018, -1.8477) construction
  line L114 (-8.018, -1.8477) -> (-7.9266, -1.9892) construction
  line L115 (-7.9266, -1.9892) -> (-7.7729, -2.0664) construction
  line L116 (-7.7729, -2.0664) -> (-7.616, -2.0664) construction
  line L117 (-7.616, -2.0664) -> (-7.5271, -2.0664) construction
  line L118 (-7.5271, -2.0664) -> (-7.4372, -2.0416) construction
  line L119 (-7.4372, -2.0416) -> (-7.357, -1.9897) construction
  line L120 (-7.357, -1.9897) -> (-7.1352, -1.8465) construction
  line L121 (-7.1352, -1.8465) -> (-7.0716, -1.5505) construction
  line L122 (-7.0716, -1.5505) -> (-7.2149, -1.3287) construction
  line L123 (-1.8239, -5.0075) -> (1.8231, -5.0075)
  constraints: 4 end point, 2 horizontal, 1 collinear, 1 point on line, 3 other
extrude "Extrusion2" cut sketch "Sketch2" against normal blind 3 contours S0 | S1 | S2 | S3
chamfer "Chamfer1" distance 3 angle 45 4 edges at (0, -44.25, 3) (-45.15, 0, 3) (0, 44.25, 3) (45.15, 0, 3)
sketch "Sketch3" plane through (0, 0, 3) normal (0, 0, 1) x (1, 0, 0)
  spline S0 degree 3 poles (9.4626, 5.1378) (9.2247, 4.9889) (9.1527, 4.6754) (9.3017, 4.4376) (9.947, 3.4071) (10.288, 2.2163) (10.288, 0.9941) (10.288, -0.2607) (9.9298, -1.4784) (9.2521, -2.5271) (9.0998, -2.7628) (9.1674, -3.0773) (9.4031, -3.2295) (9.4883, -3.2846) (9.5838, -3.3109) (9.6784, -3.3109) (9.8449, -3.3109) (10.0082, -3.229) (10.1055, -3.0786) (10.8895, -1.8651) (11.3041, -0.4568) (11.3041, 0.9941) (11.3041, 2.4073) (10.9094, 3.7845) (10.1628, 4.9769) (10.0138, 5.2146) (9.7003, 5.2867) (9.4626, 5.1378) knots 0 0 0 0 0.111111 0.111111 0.111111 0.222222 0.222222 0.222222 0.333333 0.333333 0.333333 0.444444 0.444444 0.444444 0.555556 0.555556 0.555556 0.666667 0.666667 0.666667 0.777778 0.777778 0.777778 0.888889 0.888889 0.888889 1 1 1 1 projected
  spline S1 degree 3 poles (-7.2149, -1.3287) (-7.6619, -0.6369) (-7.8981, 0.1663) (-7.8981, 0.9941) (-7.8981, 1.8005) (-7.6731, 2.5861) (-7.2474, 3.2658) (-7.1073, 3.4896) (-7.1751, 3.7846) (-7.3989, 3.9248) (-7.6227, 4.065) (-7.9177, 3.9972) (-8.0579, 3.7733) (-8.579, 2.9413) (-8.8544, 1.9803) (-8.8544, 0.9941) (-8.8544, -0.0182) (-8.5652, -1.0009) (-8.018, -1.8477) (-7.9266, -1.9892) (-7.7729, -2.0664) (-7.616, -2.0664) (-7.5271, -2.0664) (-7.4372, -2.0416) (-7.357, -1.9897) (-7.1352, -1.8465) (-7.0716, -1.5505) (-7.2149, -1.3287) knots 0 0 0 0 0.111111 0.111111 0.111111 0.222222 0.222222 0.222222 0.333333 0.333333 0.333333 0.444444 0.444444 0.444444 0.555556 0.555556 0.555556 0.666667 0.666667 0.666667 0.777778 0.777778 0.777778 0.888889 0.888889 0.888889 1 1 1 1 projected
  line L0 (-1.8239, -5.0075) -> (1.8231, -5.0075) projected
  arc A0 (-1.8239, -5.0075) -> (1.8231, -5.0075) centre (-0.0004, -4.4937) ccw projected
  spline S2 degree 3 poles (7.5776, 3.9248) (7.3538, 3.7846) (7.2861, 3.4896) (7.4262, 3.2658) (7.8519, 2.5861) (8.0769, 1.8006) (8.0769, 0.9941) (8.0769, 0.1663) (7.8407, -0.6369) (7.3937, -1.3287) (7.2504, -1.5505) (7.314, -1.8465) (7.5359, -1.9898) (7.6161, -2.0416) (7.706, -2.0664) (7.7948, -2.0664) (7.9517, -2.0664) (8.1054, -1.9892) (8.1969, -1.8476) (8.7439, -1.0008) (9.0332, -0.0181) (9.0332, 0.9941) (9.0332, 1.9804) (8.7577, 2.9414) (8.2366, 3.7734) (8.0964, 3.9972) (7.8013, 4.065) (7.5776, 3.9248) knots 0 0 0 0 0.111111 0.111111 0.111111 0.222222 0.222222 0.222222 0.333333 0.333333 0.333333 0.444444 0.444444 0.444444 0.555556 0.555556 0.555556 0.666667 0.666667 0.666667 0.777778 0.777778 0.777778 0.888889 0.888889 0.888889 1 1 1 1 projected
  spline S3 degree 3 poles (-10.1092, 0.9941) (-10.1092, 2.2164) (-9.7681, 3.4072) (-9.1228, 4.4376) (-8.9739, 4.6754) (-9.0459, 4.9889) (-9.2837, 5.1378) (-9.5216, 5.2868) (-9.835, 5.2146) (-9.9839, 4.9769) (-10.7306, 3.7846) (-11.1252, 2.4074) (-11.1252, 0.9941) (-11.1252, -0.4569) (-10.7108, -1.8652) (-9.9267, -3.0786) (-9.8295, -3.229) (-9.6662, -3.3109) (-9.4996, -3.3109) (-9.4051, -3.3109) (-9.3095, -3.2846) (-9.2243, -3.2295) (-8.9887, -3.0773) (-8.9211, -2.7628) (-9.0733, -2.5271) (-9.751, -1.4784) (-10.1092, -0.2608) (-10.1092, 0.9941) knots 0 0 0 0 0.111111 0.111111 0.111111 0.222222 0.222222 0.222222 0.333333 0.333333 0.333333 0.444444 0.444444 0.444444 0.555556 0.555556 0.555556 0.666667 0.666667 0.666667 0.777778 0.777778 0.777778 0.888889 0.888889 0.888889 1 1 1 1 projected
  line L1 (5.6617, -3.3088) -> (5.6617, -4.2334) projected
  line L2 (5.6617, -4.2334) -> (-5.6622, -4.2334) projected
  line L3 (-5.6622, -4.2334) -> (-5.6622, -3.3088) projected
  arc A1 (-4.3515, -1.9984) -> (-5.6622, -3.3088) centre (-4.3518, -3.3088) ccw projected
  line L4 (-4.3515, -1.9984) -> (-4.3515, 0.9267) projected
  arc A2 (-0.9864, 5.1508) -> (-4.3515, 0.9267) centre (-0.0178, 0.9267) ccw projected
  arc A3 (0.9967, 5.1613) -> (-0.9864, 5.1508) centre (0.0051, 5.156) ccw projected
  arc A4 (4.3515, 0.9267) -> (0.9967, 5.1613) centre (0.0016, 0.9267) ccw projected
  line L5 (4.3515, 0.9267) -> (4.3515, -1.9981) projected
  arc A5 (5.6617, -3.3088) -> (4.3515, -1.9981) centre (4.351, -3.3088) ccw projected
  line L6 (-45.15, -44.25) -> (45.15, -44.25) projected
  line L7 (45.15, 44.25) -> (-45.15, 44.25) projected
  circle A6 centre (0, 0) radius 15
  arc A7 (-5, -16.7705) -> (5, -16.7705) centre (0, 0) ccw
  line L8 (-5, 16.7705) -> (-5, 44.25)
  line L9 (5, 16.7705) -> (5, 44.25)
  line L10 (45.15, 44.25) -> (-45.15, 44.25) projected
  line L11 (-5, 44.25) -> (5, 44.25)
  line L12 (5, -16.7705) -> (5, -44.25)
  line L13 (5, -44.25) -> (-5, -44.25)
  line L14 (-5, -16.7705) -> (-5, -44.25)
  arc A8 (-5, 16.7705) -> (-5, -16.7705) centre (0, 0) ccw construction
  arc A9 (5, 16.7705) -> (-5, 16.7705) centre (0, 0) ccw
  arc A10 (5, -16.7705) -> (5, 16.7705) centre (0, 0) ccw construction
  point P0 (0, -44.25)
  dimension "d7" = 30
  dimension "d8" = 35
  dimension "d9" = 10
  constraints: 12 end point, 9 point on circle, 8 point on line, 5 centre point, 2 coincident, 2 perpendicular, 1 collinear, 1 midpoint, 1 parallel, 1 vertical alignment, 4 other
  measures "d7" diameter of A6
  measures "d8" diameter of A7
  measures "d9" distance between parallel lines of L9 L8
extrude "Extrusion3" cut sketch "Sketch3" against normal blind 1
sketch "Sketch4" plane through (0, 0, 0) normal (0, 0, -1) x (-1, 0, 0)
  line L0 (41.15, -42.75) -> (-41.15, -42.75)
  line L1 (-43.65, -40.25) -> (-43.65, 40.25)
  line L2 (-41.15, 42.75) -> (41.15, 42.75)
  line L3 (43.65, 40.25) -> (43.65, -40.25)
  line L4 (43.65, -42.75) -> (-43.65, 42.75) construction
  line L5 (-43.65, -42.75) -> (43.65, 42.75) construction
  line L6 (41.1184, -41.25) -> (-41.1184, -41.25)
  line L7 (-42.1184, -40.25) -> (-42.1184, 40.25)
  line L8 (-41.1184, 41.25) -> (41.1184, 41.25)
  line L9 (42.1184, 40.25) -> (42.1184, -40.25)
  line L10 (42.1184, -41.25) -> (-42.1184, 41.25) construction
  line L11 (-42.1184, -41.25) -> (42.1184, 41.25) construction
  arc A0 (-41.15, 42.75) -> (-43.65, 40.25) centre (-41.15, 40.25) ccw
  arc A1 (-43.65, -40.25) -> (-41.15, -42.75) centre (-41.15, -40.25) ccw
  arc A2 (41.15, -42.75) -> (43.65, -40.25) centre (41.15, -40.25) ccw
  arc A3 (43.65, 40.25) -> (41.15, 42.75) centre (41.15, 40.25) ccw
  arc A4 (-41.1184, 41.25) -> (-42.1184, 40.25) centre (-41.1184, 40.25) ccw
  arc A5 (-42.1184, -40.25) -> (-41.1184, -41.25) centre (-41.1184, -40.25) ccw
  arc A6 (41.1184, -41.25) -> (42.1184, -40.25) centre (41.1184, -40.25) ccw
  arc A7 (42.1184, 40.25) -> (41.1184, 41.25) centre (41.1184, 40.25) ccw
  line L12 (-45.15, -44.25) -> (-45.15, 44.25) projected
  line L13 (-45.15, 44.25) -> (45.15, 44.25) projected
  point P0 (-9.4626, 5.1378)
  point P1 (7.2149, -1.3287)
  point P2 (-7.5776, 3.9248)
  point P3 (10.1092, 0.9941)
  point P4 (0, 0)
  dimension "d17" = 1.5
  dimension "d18" = 2.5
  dimension "d19" = 1
  dimension "d26" = 1.5
  dimension "d27" = 1.5
  constraints: 24 end point, 17 point on line, 16 point on circle, 16 tangent, 8 centre point, 6 equal radius, 4 midpoint, 4 parallel, 2 horizontal, 2 perpendicular
  measures "d17" distance between parallel lines of L2 L8
  measures "d18" radius of A0
  measures "d19" radius of A4
  measures "d26" distance between parallel lines of L12 L1
  measures "d27" distance between parallel lines of L13 L2
extrude "Extrusion4" add sketch "Sketch4" along normal blind 8
ref_plane "Work Plane1" through (-45.15, -44.25, 0) normal (0, 1, 0) x (-1, 0, 0)
sketch "Sketch5" plane through (-45.15, -44.25, 0) normal (0, 1, 0) x (-1, 0, 0)
  line L0 (-40.15, 3) -> (-40.15, 2) projected
  line L1 (-40.15, 3) -> (-50.15, 3)
  line L2 (-50.15, 3) -> (-50.15, 0)
  line L3 (-50.15, 0) -> (-40.15, 0)
  line L4 (-40.15, 0) -> (-40.15, 3)
  line L5 (0, 0) -> (-90.3, 0) projected
  point P0 (-45.15, 0)
  constraints: 8 end point, 2 parallel, 1 coincident, 1 horizontal, 1 perpendicular, 1 point on line
extrude "Extrusion5" cut sketch "Sketch5" along normal blind 0.7
ref_plane "Work Plane2" through (-5, -43.55, 0) normal (0, -0.7071068, 0.7071068) x (1, 0, 0)
sketch "Sketch6" plane through (5, -41.25, 3) normal (0, -0.7071068, 0.7071068) x (1, 0, 0)
  line L0 (-10, 0) -> (0, 0)
  line L1 (0, 0) -> (0, -4.2426)
  line L2 (0, -4.2426) -> (-10, -4.2426)
  line L3 (-10, -4.2426) -> (-10, 0)
  point P0 (-5, 27.0468)
  constraints: 8 end point, 2 parallel, 1 horizontal, 1 perpendicular
extrude "Extrusion6" cut sketch "Sketch6" against normal up to surface (0.495 mm away)
mirror "Mirror1" about plane through (0, 0, 0) normal (0, 1, 0) of "Extrusion6"
sketch "Sketch7" plane through (43.65, -40.25, 0) normal (1, 0, 0) x (0, 0, -1)
  circle A0 centre (5, 2.75) radius 1.5
  circle A1 centre (5, 77.75) radius 1.5
  line L0 (0, -4) -> (0, 84.5) projected
  line L1 (5, 2.75) -> (5, 77.75) construction
  point P0 (0, 40.25)
  point P1 (5, 40.25)
  point P2 (0, 38.9213)
  point P3 (0, 40.25)
  dimension "d28" = 3
  dimension "d29" = 3
  dimension "d30" = 75
  dimension "d31" = 5
  constraints: 2 centre point, 2 end point, 2 midpoint, 1 horizontal alignment, 1 vertical, 1 vertical alignment
  measures "d28" diameter of A0
  measures "d29" diameter of A1
  measures "d30" distance of L1.end L1.start
  measures "d31" distance from line of L0 L1.end
extrude "Extrusion7" add sketch "Sketch7" along normal blind 1
fillet "Fillet1" radius 1 2 edges at (44.65, -37.5, -3.5) (44.65, 37.5, -3.5)
sketch "Sketch8" plane through (43.65, -40.25, 0) normal (1, 0, 0) x (0, 0, -1)
  circle A0 centre (5, 2.75) radius 1.5 projected
  line L0 (5, 1.25) -> (1.7, 1.25)
  line L1 (1.7, 1.25) -> (1.7, 0.25)
  line L2 (1.7, 0.25) -> (8, 0.25)
  line L3 (8, 0) -> (8, 80.5) projected
  line L4 (5, 4.25) -> (1.7, 4.25)
  line L5 (1.7, 4.25) -> (1.7, 5.25)
  line L6 (1.7, 5.25) -> (8, 5.25)
  line L7 (8, 5.25) -> (8, 0.25)
  line L8 (0, -4) -> (0, 84.5) projected
  circle A1 centre (5, 77.75) radius 1.5 projected
  line L9 (5, 79.25) -> (1.7, 79.25)
  line L10 (1.7, 79.25) -> (1.7, 80.25)
  line L11 (1.7, 80.25) -> (8, 80.25)
  line L12 (8, 80.25) -> (8, 75.25)
  line L13 (8, 75.25) -> (1.7, 75.25)
  line L14 (1.7, 75.25) -> (1.7, 76.25)
  line L15 (1.7, 76.25) -> (5, 76.25)
  point P0 (0, 40.25)
  dimension "d35" = 1
  dimension "d36" = 1.7
  dimension "d37" = 1.7
  dimension "d38" = 1
  dimension "d39" = 1
  dimension "d40" = 1
  dimension "d41" = 1.7
  constraints: 28 end point, 9 perpendicular, 6 point on line, 4 point on circle, 3 horizontal, 2 tangent, 2 vertical alignment
  measures "d35" distance of L0.end L1.end
  measures "d36" distance between parallel lines of L8 L1
  measures "d37" distance between parallel lines of L8 L5
  measures "d38" distance of L4.end L5.end
  measures "d39" distance of L13.end L14.end
  measures "d40" distance of L9.end L10.end
  measures "d41" distance between parallel lines of L8 L10
extrude "Extrusion8" cut sketch "Sketch8" against normal blind 1.6 contours A0 L4 L5 L6 L3 L2 L1 L0 | L13 L14 L15 A1 L9 L10 L11 L3
mirror "Mirror2" about plane through (0, 0, 0) normal (1, 0, 0) of "Extrusion8", "Fillet1", "Extrusion7"
equation "\"d37\" = d36"
equation "\"d38\" = d35"
equation "\"d39\" = d38"
equation "\"d40\" = d39"
equation "\"d41\" = d36"
body "Solid1"
